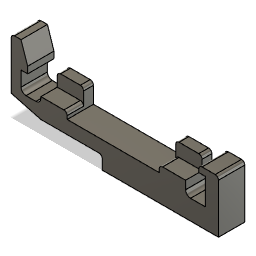
PCB_Clip v16 (Autodesk Fusion 360 design; units mm, degrees)
Autodesk Fusion 360 part; units mm, degrees
sketch "Sketch1" plane through (0, 0, 0) normal (0, 0, 1) x (1, 0, 0)
  line L0 (0, 0) -> (0, -7.7942)
  line L1 (13.8333, -11) -> (31.5, -11)
  line L2 (31.5, -11) -> (31.5, -3)
  line L3 (29.5, -4) -> (29.5, -8)
  line L4 (26.5, -6) -> (4.5, -6)
  line L5 (1.5, -7) -> (1.5, -4)
  line L6 (1.5, 0) -> (0, 0)
  line L7 (4.5, -6) -> (4.5, -7)
  line L8 (4.5, -7) -> (1.5, -7)
  line L9 (29.5, -8) -> (26.5, -8)
  line L10 (26.5, -6) -> (26.5, -8)
  line L11 (31.5, -3) -> (28.5, -3)
  line L12 (28.5, -3) -> (28.5, -4)
  line L13 (28.5, -4) -> (29.5, -4)
  line L14 (1.5, 0) -> (2.5, -3)
  line L15 (2.5, -3) -> (2.5, -4)
  line L16 (2.5, -4) -> (1.5, -4)
  line L17 (28.5, -4) -> (2.5, -4) construction
  line L18 (13.8333, -11) -> (13.8333, -9)
  line L19 (13.8333, -9) -> (4.5, -9)
  line L20 (4.5, -9) -> (0, -7.7942)
  line L21 (4.5, -7) -> (4.5, -9) construction
  dimension "d4" = 28
  dimension "d5" = 4.5
  dimension "d7" = 3
  dimension "d8" = 3
  dimension "d9" = 5
  dimension "d10" = 1
  dimension "d11" = 3
  dimension "d13" = 1
  dimension "d14" = 7
  dimension "d15" = 1
  dimension "d16" = 4
  dimension "d17" = 3
  dimension "d18" = 2.5
  dimension "d19" = 1.5
  dimension "d20" = 3
  dimension "d21" = 2
  dimension "d22" = 9.3333
  dimension "d23" = 165
  constraint coincident L0.start L6.end
  constraint vertical L0
  constraint perpendicular L0 L1
  constraint perpendicular L1 L2
  constraint perpendicular L3 L4
  constraint perpendicular L4 L5
  constraint perpendicular L0 L6
  constraint perpendicular L4 L7
  constraint perpendicular L7 L8
  constraint coincident L5.start L8.end
  constraint perpendicular L3 L9
  constraint perpendicular L9 L10
  constraint coincident L3.end L9.start
  constraint perpendicular L3 L11
  constraint perpendicular L11 L12
  constraint perpendicular L3 L13
  constraint coincident L2.end L11.start
  constraint perpendicular L6 L15
  constraint perpendicular L5 L16
  constraint horizontal L17
  constraint perpendicular L1 L18
  constraint perpendicular L18 L19
  constraint vertical L21
  measures "d4" distance of L3 L5
  measures "d5" distance of L0 L7
  measures "d7" distance of L3 L10
  measures "d8" distance of L5 L7
  measures "d9" distance of L1 L4
  measures "d10" distance of L11.end L12.end
  measures "d11" distance of L2.end L11.end
  measures "d13" distance of L12.end L3.start
  measures "d14" distance of L1 L17
  measures "d15" distance of L14.end L15.end
  measures "d16" distance of L3.end L3.start
  measures "d17" distance of L5.start L5.end
  measures "d18" distance of L0 L15
  measures "d19" distance of L6.start L0.start
  measures "d20" distance of L6 L14.end
  measures "d21" distance of L1.start L18.end
  measures "d22" distance of L18.end L19.end
  measures "d23" angle of L19 L20
extrude "Extrude1" add sketch "Sketch1" along normal blind 4
sketch "Sketch2" plane through (0, -6, 0) normal (0, 1, 0) x (-1, 0, 0)
  line L0 (-26.5, 0) -> (-4.5, 0)
  line L1 (-4.5, 0) -> (-4.5, 4)
  line L2 (-4.5, 4) -> (-26.5, 4)
  line L3 (-26.5, 4) -> (-26.5, 0)
  line L4 (-8.5, 0) -> (-22.5, 0)
  line L5 (-22.5, 0) -> (-22.5, 4)
  line L6 (-22.5, 4) -> (-8.5, 4)
  line L7 (-8.5, 4) -> (-8.5, 0)
  dimension "d31" = 14
  constraint horizontal L4
  constraint vertical L5
  constraint horizontal L6
  constraint vertical L7
  constraint coincident L2 L5.end
  constraint coincident L0 L4.start
  constraint midpoint L0 L4
  measures "d31" distance of L5 L7
extrude "Extrude2" cut sketch "Sketch2" against normal blind 1 contours L0 L2 L4 L5 L6 L7
sketch "Sketch3" plane through (0, -6, 0) normal (0, 1, 0) x (-1, 0, 0)
  line L0 (-8.5, 4) -> (-8.5, 0)
  line L1 (-8.5, 0) -> (-4.5, 0)
  line L2 (-4.5, 0) -> (-4.5, 4)
  line L3 (-4.5, 4) -> (-8.5, 4)
  line L4 (-4.5, 0) -> (-8.5, 0)
  line L5 (-8.5, 0) -> (-8.5, 1.5)
  line L6 (-8.5, 1.5) -> (-4.5, 1.5)
  line L7 (-4.5, 1.5) -> (-4.5, 0)
  dimension "d32" = 1.5
  constraint horizontal L4
  constraint vertical L5
  constraint horizontal L6
  constraint vertical L7
  constraint coincident L0 L5.end
  constraint coincident L1.end L2.start
  measures "d32" distance of L0.end L5.end
sketch "Sketch4" plane through (0, -6, 0) normal (0, 1, 0) x (-1, 0, 0)
  line L0 (-22.5, 0) -> (-22.5, 4)
  line L1 (-22.5, 4) -> (-26.5, 4)
  line L2 (-26.5, 4) -> (-26.5, 0)
  line L3 (-26.5, 0) -> (-22.5, 0)
  line L4 (-22.5, 0) -> (-26.5, 0)
  line L5 (-26.5, 0) -> (-26.5, 1.5)
  line L6 (-26.5, 1.5) -> (-22.5, 1.5)
  line L7 (-22.5, 1.5) -> (-22.5, 0)
  dimension "d33" = 1.5
  constraint horizontal L4
  constraint vertical L5
  constraint horizontal L6
  constraint vertical L7
  constraint coincident L2 L5.end
  constraint coincident L0.start L3.end
  measures "d33" distance of L0.start L6.end
extrude "Extrude3" add sketch "Sketch3" sketch "Sketch4" along normal blind 2 contours L0 L1 L2 L4 L5 L6 L7 of sketch 2 contours L0 L2 L3 L4 L5 L6 L7
fillet "Fillet1" radius 0.5 10 edges at (8.5, -4, 0.75) (8.5, -6, 2.75) (22.5, -6, 2.75) (22.5, -4, 0.75) (26.5, -4, 0.75) (4.5, -4, 0.75) (0, 0, 2) (31.5, -3, 2) (28.5, -3, 2) (13.8333, -9, 2)
fillet "Fillet1" radius 0.75 3 edges at (1.5, -7, 2) (26.5, -8, 2) (4.5, -7, 2)
equation "CLIP_PCB_SIZE = 28 mm"
equation "CLIP_PCB_THICKNESS = 2 mm"
equation "CLIP_DISTANCE_TO_BASE = 5 mm"
equation "d4 = CLIP_PCB_SIZE"
equation "d9 = CLIP_DISTANCE_TO_BASE"
equation "d14 = CLIP_DISTANCE_TO_BASE + CLIP_PCB_THICKNESS"
equation "d16 = CLIP_DISTANCE_TO_BASE + CLIP_PCB_THICKNESS - 3 mm"
equation "d17 = CLIP_DISTANCE_TO_BASE + CLIP_PCB_THICKNESS - 4 mm"
equation "d22 = CLIP_PCB_SIZE / 3"
equation "d24 = CLIP_THICKNESS"
equation "CLIP_THICKNESS = 4 mm"
equation "d31 = CLIP_PCB_SIZE - 6 mm - 6 mm - 2 mm"
